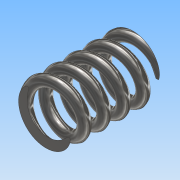
# Autodesk Inventor part: пружина
Saved by Autodesk Inventor 2017 (Build 210142000, 142)
## iProperties
Part Number: пружина
Material: Типовые
Document SubType Name: Modeling
Designer: STALKER
Density: 1 g/cm^3
Appearance: Сталь — полированная
Author: STALKER
Autodesk Inventor part; units mm, degrees
ref_plane "YZ Plane" through (0, 0, 0) normal (1, 0, 0) x (0, 1, 0)
ref_plane "XZ Plane" through (0, 0, 0) normal (0, 1, 0) x (-1, 0, 0)
ref_plane "XY Plane" through (0, 0, 0) normal (0, 0, 1) x (1, 0, 0)
sketch "Эскиз1" plane through (0, 0, 0) normal (0, 0, 1) x (1, 0, 0)
  line L0 (0, 0) -> (0, 14) construction
  circle A0 centre (2.45, 0) radius 0.55
  dimension "d0" = 1.1
  dimension "d1" = 3
  constraints: 2 end point, 1 centre point, 1 vertical
  measures "d0" diameter of A0
coil "Пружина1" sketch "Эскиз1" operation add axis through (0, 0, 0) along (0, 1, 0) pitch 2 turns 5 hand right
sketch "Эскиз2" plane through (2.45, 0, 0) normal (0, 0, 1) x (1, 0, 0)
  line L0 (-12, 19) -> (2, 19)
  line L1 (2, 19) -> (2, 9.4661)
  line L2 (2, 9.4661) -> (-12, 9.4661)
  line L3 (-12, 9.4661) -> (-12, 19)
  line L4 (-15, 0.6645) -> (13, 0.6645)
  line L5 (13, 0.6645) -> (13, -3)
  line L6 (13, -3) -> (-15, -3)
  line L7 (-15, -3) -> (-15, 0.6645)
  point P0 (-2.45, 0)
  dimension "d10" = 8.8015
  constraints: 16 end point, 4 parallel, 2 horizontal, 2 perpendicular
  measures "d10" distance between parallel lines of L4 L2
extrude "Выдавливание1" cut sketch "Эскиз2" along normal mid plane 10
